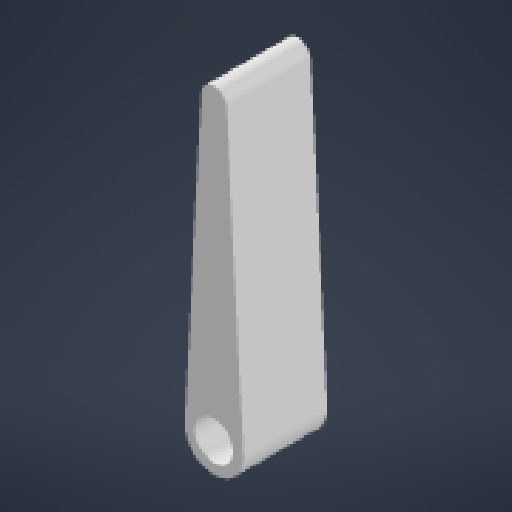
# Autodesk Inventor part: gate2
Saved by Autodesk Inventor 2026.2 (Build 302298000, 298)
## iProperties
Created: 2026-03-01
Part Number: gate2
Material: Generic
Document SubType Name: Modeling
Designer: danda
Density: 1 g/cm^3
Appearance: Default
Author: danda
Autodesk Inventor part; units mm, degrees
ref_plane "YZ Plane" through (0, 0, 0) normal (1, 0, 0) x (0, 1, 0)
ref_plane "XZ Plane" through (0, 0, 0) normal (0, 1, 0) x (-1, 0, 0)
ref_plane "XY Plane" through (0, 0, 0) normal (0, 0, 1) x (1, 0, 0)
sketch "Sketch1" plane through (0, 0, 0) normal (0, 0, 1) x (1, 0, 0)
  circle A0 centre (12.7061, -8.8819) radius 2.285
  circle A1 centre (12.7061, -8.8819) radius 3.5
  circle A2 centre (12.7061, 26.1181) radius 1.5
  line L0 (11.2061, 26.1181) -> (9.2061, -8.8819)
  line L1 (14.2061, 26.1181) -> (16.2061, -8.8819)
  point P0 (0, 0)
  dimension "d0" = 4.57
  dimension "d1" = 7
  dimension "d2" = 3
  dimension "d3" = 35
  constraints: 4 end point, 4 point on circle, 3 centre point, 1 coincident
  measures "d0" diameter of A0
  measures "d1" diameter of A1
  measures "d2" diameter of A2
  measures "d3" distance of A0.centre A2.centre
extrude "Extrusion1" add sketch "Sketch1" along normal blind 5 and the other way blind 5 contours L0 A1 L1 | L0 A2 L1 A1 | A2
body "Solid1"
